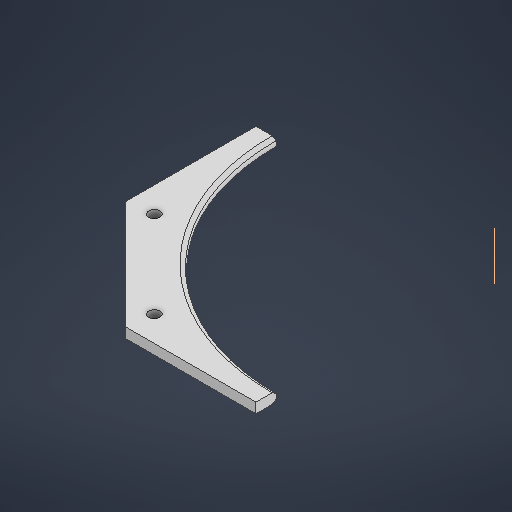
# Autodesk Inventor part: шутер на подш
Saved by Autodesk Inventor 2026.2 (Build 302298000, 298)
## iProperties
Created: 2026-01-20
Part Number: шутер на подш
Material: Типовые
Document SubType Name: Modeling
Designer: Phantom
Density: 1 g/cm^3
Appearance: По умолчанию
Author: Phantom
Autodesk Inventor part; units mm, degrees
ref_plane "YZ Plane" through (0, 0, 0) normal (1, 0, 0) x (0, 1, 0)
ref_plane "XY Plane" through (0, 0, 0) normal (0, 0, 1) x (1, 0, 0)
sketch "Эскиз1" plane through (0, 0, 0) normal (0, 0, 1) x (1, 0, 0)
  line L0 (0, 0) -> (-13, 0)
  line L1 (0, 0) -> (0, -7)
  line L2 (0, -7) -> (-13, -7)
  line L3 (0, -3.5) -> (-10, -3.5)
  arc A0 (-13, -6) -> (-13, -1) centre (-12.5417, -3.5) ccw
  arc A1 (-12.9459, -5.7049) -> (-12.9459, -1.2951) centre (-12.5417, -3.5) ccw
  line L4 (-10, -3.5) -> (-13.6021, -3.5)
  line L5 (-13.6021, -1.5) -> (-10, -1.5)
  line L6 (-10, -1.5) -> (0, -1.5)
  line L7 (-13.6021, -5.5) -> (-10, -5.5)
  line L8 (-10, -5.5) -> (0, -5.5)
  line L9 (-13.6021, -2.5) -> (-10, -2.5)
  line L10 (-10, -2.5) -> (0, -2.5)
  line L11 (-13.6021, -4.5) -> (-10, -4.5)
  line L12 (-10, -4.5) -> (0, -4.5)
  line L13 (-11.5292, -1.5) -> (-12.0292, -1.5)
  line L14 (-12.0292, -1.5) -> (-10.5354, -2.5)
  line L15 (-12.0292, -5.5) -> (-10.5354, -4.5)
  line L16 (-13.6021, -1.5) -> (-13.6021, -5.5)
  point P0 (-10.5354, -4.5)
  dimension "d0" = 13
  dimension "d1" = 7
  dimension "d2" = 1
  dimension "d3" = 1
  dimension "d4" = 10
  dimension "d5" = 0.3
  dimension "d6" = 2
  dimension "d7" = 2
  dimension "d8" = 1
  dimension "d9" = 1
  dimension "d10" = 0.5
  constraints: 34 end point, 7 point on circle, 3 horizontal, 3 point on line, 2 centre point, 2 symmetric about line, 2 vertical, 1 midpoint, 1 perpendicular, 4 other
  measures "d0" distance of L0.start L0.end
  measures "d1" distance of L0.start L1.end
  measures "d2" distance of L2.end A0.start
  measures "d3" distance of L0.end A0.end
  measures "d4" distance of L3.start L3.end
  measures "d5" radial gap between concentric circles of A0 A1
  measures "d6" distance between parallel lines of L4 L5
  measures "d7" distance between parallel lines of L4 L7
  measures "d8" distance between parallel lines of L4 L9
  measures "d9" distance between parallel lines of L4 L11
  measures "d10" distance of L13.start L13.end
sketch "Эскиз2" plane through (0, 0, 0) normal (0, 1, 0) x (-1, 0, 0)
  line L0 (13, 0) -> (10, 0) projected
  line L1 (10, 0) -> (-76.5, 0)
  circle A0 centre (-76.5, 0) radius 86.5
  point P0 (0, 0)
  dimension "d13" = 86.5
  constraints: 2 end point, 1 coincident, 1 horizontal, 1 horizontal alignment, 2 other
  measures "d13" distance of L0.end L1.end
sweep "Сдвиг1" add profiles "Эскиз1" path "Эскиз2" path curves A0 contours L4 L16 L9 A1 | A1 L11 L16 L4 | L9 L16 L5 L14 | L15 L7 L16 L11
sketch "Эскиз3" plane through (0, 0, 0) normal (0, 1, 0) x (-1, 0, 0)
  circle A0 centre (-76.5, 0) radius 90.1021 projected
  line L0 (18.5, -95) -> (-171.5, -95)
  line L1 (-171.5, -95) -> (-171.5, 95)
  line L2 (-171.5, 95) -> (18.5, 95)
  line L3 (18.5, 95) -> (18.5, -95)
  line L4 (18.5, -95) -> (-171.5, 95) construction
  line L5 (-171.5, -95) -> (18.5, 95) construction
  circle A1 centre (-76.5, 0) radius 87.0354 projected
  point P0 (0, 0)
  dimension "d16" = 190
  dimension "d17" = 190
  constraints: 12 end point, 2 midpoint, 2 parallel, 1 horizontal, 1 perpendicular
  measures "d16" distance of L1.end L2.end
  measures "d17" distance of L0.end L1.end
extrude "Выдавливание2" add sketch "Эскиз3" against normal up to surface (5.5 mm away) contours L0 L1 L2 L3
sketch "Эскиз4" plane through (0, 0, 0) normal (0, 1, 0) x (1, 0, 0)
  line L0 (-18.5, -95) -> (171.5, -95) projected
  line L1 (171.5, -95) -> (171.5, 95) projected
  line L2 (171.5, 95) -> (-18.5, 95) projected
  line L3 (-18.5, 95) -> (-18.5, -95) projected
  circle A0 centre (76.5, 0) radius 90.1021 projected
  point P0 (0, 0)
extrude "Выдавливание3" cut sketch "Эскиз4" against normal up to surface (1.5 mm away)
sketch "Эскиз5" plane through (-18.5, -1.5, -95) normal (0, 1, 0) x (1, 0, 0)
  line L0 (0, 0) -> (190, 0) projected
  line L1 (0, -190) -> (0, 0) projected
  line L2 (190, -190) -> (0, -190) projected
  line L3 (190, 0) -> (190, -190) projected
  circle A0 centre (95, -95) radius 88.5292 projected
  line L4 (0, -146.7657) -> (43.2343, -190)
  line L5 (32.4004, -157.5996) -> (21.6172, -168.3828)
  line L6 (0, -135.452) -> (54.548, -190)
  circle A1 centre (10.0514, -145.5033) radius 2.25
  circle A2 centre (44.4967, -179.9486) radius 2.25
  point P0 (18.5, -95)
  dimension "d22" = 45
  dimension "d24" = 8
  dimension "d26" = 4.5
  dimension "d34" = 95.779
  dimension "d41" = 24.3565
  constraints: 6 end point, 5 point on line, 2 centre point, 1 midpoint, 1 parallel, 1 symmetric about line, 4 other
  measures "d22" angle of L4 L1
  measures "d24" distance between parallel lines of L4 L6
  measures "d26" diameter of A1
  measures "d34" distance from line of point (95, -95) L6
  measures "d41" distance from line of L5 A1.centre
extrude "Выдавливание4" cut sketch "Эскиз5" against normal blind 10 contours L4 L2 L1 | A1 L6 | L6 A1 | A2 L6 | L6 A2
sketch "Эскиз6" plane through (24.7343, -1.5, 95) normal (0, 1, 0) x (1, 0, 0)
  line L0 (-43.2343, 190) -> (-43.2343, 43.2343) projected
  line L1 (146.7657, 190) -> (146.7657, 0) projected
  line L2 (-43.2343, 190) -> (146.7657, 190) projected
  line L3 (146.7657, 0) -> (0, 0) projected
  line L4 (-43.2343, 43.2343) -> (-43.2343, 190) projected
  line L5 (-43.2343, 43.2343) -> (0, 0) projected
  line L6 (146.7657, 0) -> (0, 0) projected
  line L7 (146.7657, 190) -> (146.7657, 0) projected
  line L8 (-43.2343, 190) -> (146.7657, 190) projected
  circle A0 centre (-33.183, 44.4967) radius 2.25 projected
  circle A1 centre (51.7657, 95) radius 88.5292 projected
  line L9 (-43.2343, 95) -> (146.7657, 95)
  line L10 (51.7657, 0) -> (51.7657, 190)
  point P0 (-24.7343, 95)
  point P1 (-43.2343, 116.6172)
  point P2 (-57.5775, 152.4225)
  point P3 (152.4225, 152.4225)
  point P4 (152.4225, 57.5775)
  point P5 (0, 210)
  point P6 (94.845, 210)
  point P7 (73.3828, 0)
  point P8 (94.845, 0)
  point P9 (0, 0)
  point P10 (51.7657, 95)
  constraints: 4 end point, 3 midpoint, 2 point on line, 4 other
extrude "Выдавливание5" cut sketch "Эскиз6" against normal blind 10 contours L2 L10 A1 L9 L0 | L2 L1 L9 A1 L10 | A1 L10 L9 | A1 L9 L10 | L10 L9 A1 | A1 L9 L1 L3 L10 picked at (-6.9534, 99.1997) picked at (98.8928, 130.2789) picked at (93.3924, 53.3733)
